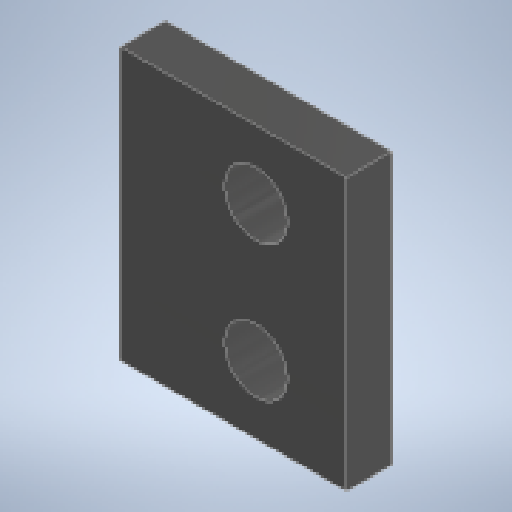
# Autodesk Inventor part: HCMUTE-CDT23-DE_CHEM_LOADCELL
Saved by Autodesk Inventor 2023 (Build 270158000, 158)
## iProperties
Created: 2023-10-14
Part Number: HCMUTE-CDT23-DE_CHEM_LOADCELL
Material: PMMA Plastic
Document SubType Name: Modeling
Designer: havie
Density: 1.188 g/cm^3
Appearance: Dark Gray
Author: havie
Autodesk Inventor part; units mm, degrees
ref_plane "YZ Plane" through (0, 0, 0) normal (1, 0, 0) x (0, 1, 0)
ref_plane "XZ Plane" through (0, 0, 0) normal (0, 1, 0) x (-1, 0, 0)
ref_plane "XY Plane" through (0, 0, 0) normal (0, 0, 1) x (1, 0, 0)
sketch "Sketch1" plane through (0, 0, 0) normal (0, 0, 1) x (1, 0, 0)
  line L0 (-12.5, -15) -> (12.5, -15)
  line L1 (12.5, -15) -> (12.5, 15)
  line L2 (12.5, 15) -> (-12.5, 15)
  line L3 (-12.5, 15) -> (-12.5, -15)
  line L4 (-12.5, -15) -> (12.5, 15) construction
  line L5 (12.5, -15) -> (-12.5, 15) construction
  point P0 (0, 0)
  dimension "d0" = 30
  dimension "d1" = 25
  constraints: 12 end point, 2 midpoint, 2 parallel, 1 horizontal, 1 perpendicular
  measures "d0" distance of L2.end L0.start
  measures "d1" distance of L0.start L0.end
extrude "Extrusion1" add sketch "Sketch1" along normal mid plane 5
sketch "Sketch2" plane through (0, 0, 2.5) normal (0, 0, 1) x (1, 0, 0)
  line L0 (-12.5, 15) -> (-12.5, -15) projected
  line L1 (12.5, 15) -> (-12.5, 15) projected
  point P0 (0, 0)
  point P1 (2.5, 7.5)
  point P2 (2.5, -7.5)
  dimension "d4" = 15
  dimension "d5" = 7.5
  dimension "d6" = 15
  constraints: 1 vertical alignment
  measures "d4" distance from line of L0 point (2.5, 7.5)
  measures "d5" distance from line of L1 point (2.5, 7.5)
  measures "d6" distance of point (2.5, -7.5) point (2.5, 7.5)
hole "Hole1" at (2.5, 7.5, 2.5) at (2.5, -7.5, 2.5) direction (0, 0, -1) diameter 7 depth 14.2 tip angle 118
body "Solid1"
